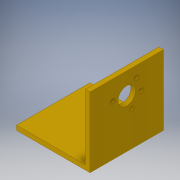
# Autodesk Inventor part: MotorMount
Saved by Autodesk Inventor 2017 (Build 210142000, 142)
## iProperties
Created: 2017-02-08
Part Number: MotorMount
Material: Generic
Document SubType Name: Modeling
Designer: Joseph
Density: 1 g/cm^3
Appearance: Gold
Author: Joseph
Autodesk Inventor part; units mm, degrees
ref_plane "YZ Plane" through (0, 0, 0) normal (1, 0, 0) x (0, 1, 0)
ref_plane "XZ Plane" through (0, 0, 0) normal (0, 1, 0) x (-1, 0, 0)
ref_plane "XY Plane" through (0, 0, 0) normal (0, 0, 1) x (1, 0, 0)
sketch "Sketch1" plane through (0, 0, 0) normal (0, 0, 1) x (1, 0, 0)
  line L0 (0, 0) -> (0, 1.5875)
  line L1 (0, 1.5875) -> (23.8125, 1.5875)
  line L2 (23.8125, 1.5875) -> (23.8125, 24.2075)
  line L3 (23.8125, 24.2075) -> (25.4, 24.2075)
  line L4 (25.4, 24.2075) -> (25.4, 0)
  line L5 (25.4, 0) -> (0, 0)
  dimension "d0" = 1.5875
  dimension "d3" = 90
  dimension "d9" = 25.4
  dimension "d10" = 22.62
  constraints: 12 end point, 6 perpendicular, 1 vertical
  measures "d0" distance of L0.start L0.end
  measures "d3" angle of L2 L1
  measures "d9" distance of L4.end L0.start
  measures "d10" distance of L1.end L2.end
extrude "Extrusion1" add sketch "Sketch1" along normal blind 25.4
sketch "Sketch2" plane through (25.4, 0, 0) normal (1, 0, 0) x (0, 0, -1)
  circle A0 centre (-12.7, 16.7075) radius 7.5
  line L0 (0, 24.2075) -> (-25.4, 24.2075) projected
  circle A1 centre (-12.7, 16.7075) radius 5
  line L1 (-12.7, 16.7075) -> (-9.4861, 20.5377)
  line L2 (-12.7, 16.7075) -> (-7.776, 15.8393)
  line L3 (-12.7, 16.7075) -> (-10.9899, 12.009)
  line L4 (-12.7, 16.7075) -> (-17.624, 17.5757)
  line L5 (-25.4, 0) -> (-25.4, 24.2075) projected
  point P0 (0, 0)
  dimension "d6" = 12.7
  dimension "d7" = 7.5
  dimension "d8" = 15
  dimension "d11" = 10
  dimension "d12" = 40
  dimension "d13" = 60
  dimension "d14" = 60
  dimension "d15" = 120
  constraints: 8 end point, 4 point on circle, 2 centre point, 1 coincident
  measures "d6" horizontal distance of point (0, 0) A0.centre
  measures "d7" distance from line of A0.centre L0
  measures "d8" diameter of A0
  measures "d11" diameter of A1
  measures "d12" angle of L5 L1
  measures "d13" angle of L2 L1
  measures "d14" angle of L3 L2
  measures "d15" angle of L1 L4
hole "Hole1" at (25.4, 17.5757, 17.624) at (25.4, 20.5377, 9.4861) at (25.4, 15.8393, 7.776) at (25.4, 12.009, 10.9899) direction (-1, 0, 0) diameter 1.5 end through all
sketch "Sketch3" plane through (25.4, 0, 0) normal (1, 0, 0) x (0, 0, -1)
  circle A0 centre (-12.7, 16.7075) radius 7.5
  line L0 (0, 24.2075) -> (-25.4, 24.2075) projected
  line L1 (0, 24.2075) -> (0, 0) projected
  dimension "d23" = 15
  dimension "d24" = 7.5
  dimension "d25" = 12.7
  constraints: 1 centre point
  measures "d23" diameter of A0
  measures "d24" distance from line of L0 A0.centre
  measures "d25" distance from line of L1 A0.centre
hole "Hole2" at (25.4, 16.7075, 12.7) direction (-1, 0, 0) diameter 6 end through all
body "Solid1"
